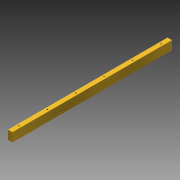
# Autodesk Inventor part: mounting rail 9.0 x.250 x.500-B
Saved by Autodesk Inventor 2013 (Build 170138000, 138)
## iProperties
Created: 2014-01-27
Part Number: mounting rail 9.0 x.250 x.500-B
Material: Gold
Document SubType Name: Modeling
Designer: rtreacy
Density: 1 g/cm^3
Author: rtreacy
Autodesk Inventor part; units mm, degrees
ref_plane "YZ Plane" through (0, 0, 0) normal (1, 0, 0) x (0, 1, 0)
ref_plane "XZ Plane" through (0, 0, 0) normal (0, 1, 0) x (-1, 0, 0)
ref_plane "XY Plane" through (0, 0, 0) normal (0, 0, 1) x (1, 0, 0)
sketch "Sketch2" plane through (0, 0, 0) normal (0, 0, 1) x (1, 0, 0)
  line L0 (-8.2799, 8.6846) -> (-1.9299, 8.6846)
  line L1 (-1.9299, 8.6846) -> (-1.9299, -4.0154)
  line L2 (-1.9299, -4.0154) -> (-8.2799, -4.0154)
  line L3 (-8.2799, -4.0154) -> (-8.2799, 8.6846)
  point P0 (0, 0)
  dimension "d3" = 6.35
  dimension "d5" = 12.7
  constraints: 8 end point, 2 parallel, 1 horizontal, 1 perpendicular
  measures "d3" distance of L0.start L0.end
  measures "d5" distance of L2.end L0.start
extrude "Extrusion1" add sketch "Sketch2" along normal blind 228.6
sketch "Sketch3" plane through (-1.9299, -4.0154, 0) normal (1, 0, 0) x (0, 0, -1)
  point P0 (-228.6, 12.7)
  point P1 (0, 4.0154)
  point P2 (-210.82, 3.2944)
  point P3 (-20.32, 3.2944)
  dimension "d8" = 9.4056
  dimension "d9" = 17.78
  dimension "d60" = 208.28
  dimension "d61" = 9.4056
  measures "d8" vertical distance of point (-228.6, 12.7) point (-210.82, 3.294)
  measures "d9" horizontal distance of point (-228.6, 12.7) point (-210.82, 3.294)
  measures "d60" horizontal distance of point (-228.6, 12.7) point (-20.32, 3.294)
  measures "d61" vertical distance of point (-228.6, 12.7) point (-20.32, 3.294)
hole "Hole1" at (-1.9299, -0.7211, 210.82) direction (-1, 0, 0) diameter 1.7018 end through all
pattern_linear "Rectangular Pattern1" count 4 spacing 25.4 along (0, 0, -1) of "Hole1"
hole "Hole5" at (-1.9299, -0.7211, 20.32) direction (-1, 0, 0) diameter 1.7018 end through all
sketch "Sketch7" plane through (-8.2799, 8.6846, 0) normal (0, 1, 0) x (1, 0, 0)
  point P0 (6.35, -228.6)
  point P1 (8.2799, 0)
  point P2 (3.175, -215.9)
  dimension "d69" = 12.7
  dimension "d70" = 3.175
  measures "d69" vertical distance of point (6.35, -228.6) point (3.175, -215.9)
  measures "d70" horizontal distance of point (6.35, -228.6) point (3.175, -215.9)
hole "Hole6" at (-5.1049, 8.6846, 215.9) direction (0, -1, 0) diameter 1.7018 depth 6.35 tip angle 118
pattern_linear "Rectangular Pattern5" count 6 spacing 40.64 along (0, 0, -1) of "Hole6"
body "Solid1"
